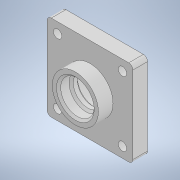
# Autodesk Inventor part: Motor to Bearing Adapter
Saved by Autodesk Inventor 2022 (Build 260153000, 153)
## iProperties
Created: 2022-03-26
Part Number: Motor to Bearing Adapter
Material: Generic
Document SubType Name: Modeling
Designer: Nick
Density: 1 g/cm^3
Appearance: Default
Author: Nick
Autodesk Inventor part; units mm, degrees
ref_plane "YZ Plane" through (0, 0, 0) normal (1, 0, 0) x (0, 1, 0)
ref_plane "XZ Plane" through (0, 0, 0) normal (0, 1, 0) x (-1, 0, 0)
ref_plane "XY Plane" through (0, 0, 0) normal (0, 0, 1) x (1, 0, 0)
sketch "Sketch1" plane through (0, 0, 0) normal (0, 0, 1) x (1, 0, 0)
  line L0 (5, 36) -> (36, 36) construction
  line L1 (36, 36) -> (36, 5) construction
  line L2 (36, 5) -> (5, 5) construction
  line L3 (5, 5) -> (5, 36) construction
  line L4 (41, 41) -> (0, 41)
  line L5 (0, 41) -> (0, 0)
  line L6 (0, 0) -> (41, 0)
  line L7 (41, 0) -> (41, 41)
  dimension "d0" = 31
  dimension "d1" = 5
  constraints: 16 end point, 4 coincident, 4 parallel, 3 perpendicular, 1 horizontal, 3 other
  measures "d0" distance of L1.end L2.end
  measures "d1" distance between parallel lines of L0 L4
extrude "Extrusion1" add sketch "Sketch1" along normal blind 7
hole "Hole1" at (5, 36, 0) at (36, 36, 0) at (36, 5, 0) at (5, 5, 0) direction (0, 0, 1) diameter 4 end through all
sketch "Sketch2" plane through (0, 0, 7) normal (0, 0, 1) x (1, 0, 0)
  circle A0 centre (20.5, 20.5) radius 11
  circle A1 centre (20.5, 20.5) radius 8 construction
  line L0 (41, 0) -> (41, 41) projected
  line L1 (41, 41) -> (0, 41) projected
  point P0 (0, 0)
  point P1 (41, 20.5)
  point P2 (20.5, 41)
  dimension "d11" = 22
  dimension "d12" = 16
  constraints: 2 centre point, 2 midpoint, 1 coincident, 1 horizontal alignment, 1 vertical alignment
  measures "d11" diameter of A0
  measures "d12" diameter of A1
extrude "Extrusion2" add sketch "Sketch2" along normal blind 7
sketch "Sketch3" plane through (20.5, 20.5, 14) normal (0, 0, 1) x (1, 0, 0)
  circle A0 centre (0, 0) radius 11 projected
  circle A1 centre (0, 0) radius 8
  point P0 (-20.5, -20.5)
  dimension "d15" = 16
  constraints: 1 centre point, 1 coincident
  measures "d15" diameter of A1
extrude "Extrusion3" cut sketch "Sketch3" against normal through all contours A1
ref_plane "Work Plane1" through (0, 0, 7) normal (0, 0, -1) x (-1, 0, 0)
sketch "Sketch4" plane through (0, 0, 7) normal (0, 0, -1) x (-1, 0, 0)
  circle A0 centre (-20.5, 20.5) radius 8 projected
  circle A1 centre (-20.5, 20.5) radius 11 projected
  circle A2 centre (-20.5, 20.5) radius 7
  point P0 (0, 0)
  dimension "d18" = 1
  constraints: 1 centre point
  measures "d18" radial gap between concentric circles of A0 A2
extrude "Extrusion4" add sketch "Sketch4" along normal mid plane 4 contours A0
chamfer "Chamfer1" distance 1 angle 45 2 edges at (27.5, 20.5, 9) (27.5, 20.5, 5)
fillet "Fillet1" radius 2 4 edges at (0, 41, 3.5) (0, 0, 3.5) (41, 0, 3.5) (41, 41, 3.5)
chamfer "Chamfer2" distance 1 angle 45 2 edges at (12.5, 20.5, 0) (12.5, 20.5, 14)
body "Solid1"
